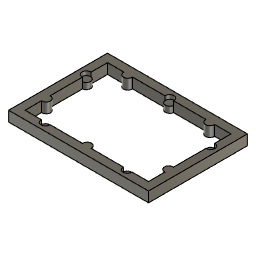
grove_3x2_sensor_mount (Autodesk Fusion 360 design; units mm, degrees)
Autodesk Fusion 360 part; units mm, degrees
sketch "Sketch2" plane through (0, 0, 0) normal (0, 0, 1) x (-1, 0, 0)
  line L0 (-34, 24) -> (-34, -24)
  line L1 (-34, -24) -> (34, -24)
  line L2 (34, -24) -> (34, 24)
  line L3 (34, 24) -> (-34, 24)
  line L4 (34.1, 24.1) -> (-34.1, 24.1)
  line L5 (-34.1, 24.1) -> (-34.1, -24.1)
  line L6 (-34.1, -24.1) -> (34.1, -24.1)
  line L7 (34.1, -24.1) -> (34.1, 24.1)
  line L8 (34.1, 24.1) -> (-34.1, -24.1) construction
  line L9 (-34.1, 24.1) -> (34.1, -24.1) construction
  dimension "d5" = 68.2
  dimension "d6" = 48.2
  constraint horizontal L4
  constraint perpendicular L4 L5
  constraint parallel L4 L6
  constraint parallel L5 L7
  constraint coincident L8 origin
  constraint coincident L9 origin
  measures "d5" distance of L5.end L6.end
  measures "d6" distance of L4.end L5.end
extrude "Extrude2" add sketch "Sketch2" along normal blind 5 contours L0 L1 L2 L3 | L4 L5 L6 L7
shell "Shell1" thickness 4 removed faces 2 at (11.3667, 8.0333, 0) at (11.3667, 8.0333, 5)
sketch "pillar sketch" plane through (0, 0, 5) normal (0, 0, 1) x (-1, 0, 0)
  line L0 (30.1, -20.1) -> (-30.1, -20.1)
  line L1 (-30.1, -20.1) -> (-30.1, 20.1)
  line L2 (-30.1, 20.1) -> (30.1, 20.1)
  line L3 (30.1, 20.1) -> (30.1, -20.1)
  line L4 (34.1, -24.1) -> (34.1, 24.1)
  line L5 (34.1, 24.1) -> (-34.1, 24.1)
  line L6 (-34.1, 24.1) -> (-34.1, -24.1)
  line L7 (-34.1, -24.1) -> (34.1, -24.1)
  circle A0 centre (0, 19.9) radius 2.1
  circle A1 centre (29.9, 10) radius 2.1
  circle A2 centre (-29.9, 10) radius 2.1
  circle A3 centre (20, -19.9) radius 2.1
  circle A4 centre (-20, -19.9) radius 2.1
  dimension "d11" = 4.2
  dimension "d15" = 4.2
  dimension "d18" = 4.2
  dimension "d23" = 0.2
  dimension "d24" = 0.2
  dimension "d25" = 0.2
  dimension "d27" = 4.2
  dimension "d28" = 0.2
  dimension "d29" = 10.1
  dimension "d30" = 10.1
  dimension "d31" = 10.1
  dimension "d32" = 4.2
  dimension "d33" = 0.2
  dimension "d34" = 10.1
  measures "d11" diameter of A0
  measures "d15" diameter of A1
  measures "d18" diameter of A2
  measures "d23" distance of L3 A1.centre
  measures "d24" distance of L2 A0.centre
  measures "d25" distance of L1 A2.centre
  measures "d27" diameter of A3
  measures "d28" distance of L0 A3.centre
  measures "d29" distance of L3 A3.centre
  measures "d30" distance of L2 A1.centre
  measures "d31" distance of L2 A2.centre
  measures "d32" diameter of A4
  measures "d33" distance of L0 A4.centre
  measures "d34" distance of L1 A4.centre
extrude "Extrude3" add sketch "pillar sketch" against normal blind 5 contours L0 A3 | L3 A1 | L0 A4 | L2 A0 | L1 A2 picked at (20.5146, -19.3943) picked at (29.3788, 9.752) picked at (-19.3838, -19.1714) picked at (0.6581, 19.0774) picked at (-29.3932, 10.2832)
sketch "hollow sketch A" plane through (0, 0, 5) normal (0, 0, 1) x (-1, 0, 0)
  line L0 (30.1, -20.1) -> (22.0905, -20.1)
  arc A0 (22.0905, -20.1) -> (17.9095, -20.1) centre (20, -19.9) ccw
  line L1 (17.9095, -20.1) -> (-17.9095, -20.1)
  arc A1 (-17.9095, -20.1) -> (-22.0905, -20.1) centre (-20, -19.9) ccw
  line L2 (-22.0905, -20.1) -> (-30.1, -20.1)
  line L3 (-30.1, -20.1) -> (-30.1, 7.9095)
  arc A2 (-30.1, 7.9095) -> (-30.1, 12.0905) centre (-29.9, 10) ccw
  line L4 (-30.1, 12.0905) -> (-30.1, 20.1)
  line L5 (-30.1, 20.1) -> (-2.0905, 20.1)
  arc A3 (-2.0905, 20.1) -> (2.0905, 20.1) centre (0, 19.9) ccw
  line L6 (2.0905, 20.1) -> (30.1, 20.1)
  line L7 (30.1, 20.1) -> (30.1, 12.0905)
  arc A4 (30.1, 12.0905) -> (30.1, 7.9095) centre (29.9, 10) ccw
  line L8 (30.1, 7.9095) -> (30.1, -20.1)
  line L9 (34.1, -24.1) -> (34.1, 24.1)
  line L10 (34.1, 24.1) -> (-34.1, 24.1)
  line L11 (-34.1, 24.1) -> (-34.1, -24.1)
  line L12 (-34.1, -24.1) -> (34.1, -24.1)
  circle A5 centre (20, 20.3) radius 2.1
  circle A6 centre (30.3, -10) radius 2.1
  circle A7 centre (-30.3, -10) radius 2.1
  circle A8 centre (0, -20.3) radius 2.1
  circle A9 centre (-20, 20.3) radius 2.1
  dimension "d37" = 4.2
  dimension "d38" = 4.2
  dimension "d39" = 4.2
  dimension "d40" = 4.2
  dimension "d41" = 4.2
  dimension "d42" = 0.2
  dimension "d44" = 0.2
  dimension "d45" = 10.1
  dimension "d46" = 10.1
  dimension "d47" = 10.1
  dimension "d49" = 10.1
  dimension "d51" = 0.2
  measures "d37" diameter of A5
  measures "d38" diameter of A6
  measures "d39" diameter of A7
  measures "d40" diameter of A8
  measures "d41" diameter of A9
  measures "d42" distance of L1 A8.centre
  measures "d44" distance of L3 A7.centre
  measures "d45" distance of L2 A7.centre
  measures "d46" distance of L0 A6.centre
  measures "d47" distance of L7 A5.centre
  measures "d49" distance of L4 A9.centre
  measures "d51" distance of L5 A9.centre
extrude "Extrude4" add sketch "hollow sketch A" against normal blind 3 from surface at -2 contours L8 A6 | L1 A8 | L6 A5 | L3 A7 | L5 A9 picked at (29.4743, -9.8971) picked at (-0.2209, -19.3952) picked at (20.5114, 18.7272) picked at (-28.7439, -10.2036) picked at (-20.6202, 19.3298)
extrude "Extrude5" cut sketch "hollow sketch A" against normal blind 2 contours L8 A6 | L1 A8 | L1 A8 | L6 A5 | L6 A5 | L3 A7 | L3 A7 | L5 A9 | L5 A9 picked at (30.8398, -9.8081)
equation "d5 = 68 mm + space_error * 2"
equation "d6 = 48 mm + space_error * 2"
equation "error_hollow = 0.2 mm" comment "das wo e ussparig isch, grechnet vom innere rand"
equation "d11 = diam_pillar"
equation "diam_hollow = 4.2 mm" comment "das wo e ussparig isch, dr durchmesser"
equation "error_pillar = 0.2 mm" comment "das wo ine e sühle isch, grechnet vom innere rand"
equation "diam_pillar = 4.2 mm" comment "das wo ine e sühle isch, dr durchmesser"
equation "d15 = diam_pillar"
equation "d18 = diam_pillar"
equation "d23 = error_pillar"
equation "d24 = error_pillar"
equation "d25 = error_pillar"
equation "d27 = diam_pillar"
equation "d28 = error_pillar"
equation "d29 = 10 mm + space_error"
equation "d30 = 10 mm + space_error"
equation "d31 = 10 mm + space_error"
equation "d32 = diam_pillar"
equation "d33 = error_pillar"
equation "d34 = 10 mm + space_error"
equation "d37 = diam_hollow"
equation "d38 = diam_hollow"
equation "d39 = diam_hollow"
equation "d40 = diam_hollow"
equation "d41 = diam_hollow"
equation "d42 = error_hollow"
equation "d44 = error_hollow"
equation "d45 = 10 mm + space_error"
equation "d46 = 10 mm + space_error"
equation "d47 = 10 mm + space_error"
equation "space_error = 0.1 mm"
equation "d49 = 10 mm + space_error"
equation "d50 = -error_hollow"
equation "d51 = error_hollow"
equation "d66 = -error_hollow"
